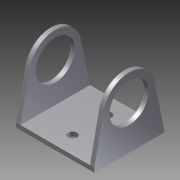
# Autodesk Inventor part: shooter bearing bracket
Saved by Autodesk Inventor 2012 (Build 160160000, 160)
## iProperties
Created: 2013-07-07
Part Number: shooter bearing bracket
Material: Default
Document SubType Name: Modeling
Designer: Bryce
Density: 1 g/cm^3
Author: Bryce
Autodesk Inventor part; units mm, degrees
ref_plane "YZ Plane" through (0, 0, 0) normal (1, 0, 0) x (0, 1, 0)
ref_plane "XZ Plane" through (0, 0, 0) normal (0, 1, 0) x (-1, 0, 0)
ref_plane "XY Plane" through (0, 0, 0) normal (0, 0, 1) x (1, 0, 0)
sketch "Sketch1" plane through (0, 0, 0) normal (0, 0, 1) x (1, 0, 0)
  line L0 (0, 0) -> (57.15, 0)
  line L1 (57.15, 0) -> (57.15, 50.8)
  line L2 (0, 50.8) -> (0, 0)
  line L3 (53.975, 50.8) -> (53.975, 3.175)
  line L4 (53.975, 3.175) -> (3.175, 3.175)
  line L5 (3.175, 3.175) -> (3.175, 50.8)
  line L6 (0, 50.8) -> (3.175, 50.8)
  line L7 (53.975, 50.8) -> (57.15, 50.8)
  dimension "d0" = 50.8
  dimension "d1" = 57.15
  dimension "d2" = 3.175
  dimension "d3" = 3.175
  dimension "d4" = 3.175
  constraints: 16 end point, 3 equal length, 2 perpendicular, 1 horizontal, 1 horizontal alignment
  measures "d0" distance of L0.end L1.end
  measures "d1" distance of L0.start L0.end
  measures "d2" distance between parallel lines of L0 L4
  measures "d3" distance between parallel lines of L2 L5
  measures "d4" distance between parallel lines of L1 L3
extrude "Extrusion1" add sketch "Sketch1" along normal blind 50.8
sketch "Sketch2" plane through (57.15, 0, 0) normal (1, 0, 0) x (0, 0, -1)
  line L0 (-50.8, 50.8) -> (-50.8, 0) projected
  line L1 (0, 0) -> (0, 50.8) projected
  line L2 (0, 50.8) -> (-50.8, 50.8) projected
  line L3 (0, 3.175) -> (-50.8, 3.175) projected
  circle A0 centre (-25.4, 31.75) radius 14.2875
  arc A1 (-6.749, 35.6286) -> (-44.051, 35.6286) centre (-25.4, 31.75) ccw
  line L4 (-44.051, 35.6286) -> (-50.8, 3.175)
  line L5 (-6.749, 35.6286) -> (0, 3.175)
  dimension "d7" = 28.575
  dimension "d8" = 25.4
  dimension "d9" = 19.05
  constraints: 4 end point, 3 tangent, 2 centre point, 2 point on circle, 1 coincident
  measures "d7" diameter of A0
  measures "d8" distance from line of L0 A0.centre
  measures "d9" distance from line of L2 A0.centre
extrude "Extrusion2" cut sketch "Sketch2" against normal through all contours L2 A1 L4 L0 | L2 L1 L5 A1 | A0
sketch "Sketch3" plane through (3.175, 3.175, 50.8) normal (0, 1, 0) x (1, 0, 0)
  line L0 (0, 0) -> (50.8, 0) projected
  line L1 (50.8, 50.8) -> (50.8, 0) projected
  line L2 (50.8, 50.8) -> (0, 50.8) projected
  circle A0 centre (25.4, 38.1) radius 3.175
  circle A1 centre (25.4, 12.7) radius 3.175
  line L3 (0, 50.8) -> (0, 0) projected
  point P0 (-3.175, 50.8)
  dimension "d12" = 6.35
  dimension "d13" = 6.35
  dimension "d14" = 12.7
  dimension "d15" = 25.4
  dimension "d16" = 12.7
  dimension "d17" = 25.4
  dimension "d20" = 50.8
  constraints: 2 centre point
  measures "d12" diameter of A0
  measures "d13" diameter of A1
  measures "d14" distance from line of L2 A0.centre
  measures "d15" distance from line of L1 A0.centre
  measures "d16" distance from line of L0 A1.centre
  measures "d17" distance from line of L1 A1.centre
  measures "d20" distance between parallel lines of L1 L3
extrude "Extrusion3" cut sketch "Sketch3" against normal blind 50.8 contours A0 | A1
equation "\"d3\" = d2"
equation "\"d4\" = d2"
equation "\"d12\" = d13"
equation "\"d15\" = 0.5 * d20"
equation "\"d16\" = d14"
equation "\"d17\" = d15"
body "Solid1"
